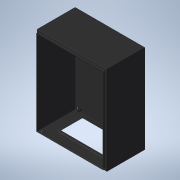
# Autodesk Inventor part: 1376.000(1)_P1
Saved by Autodesk Inventor 2021 (Build 250183000, 183)
## iProperties
Created: 2025-05-05
Part Number: 1376.000(1)_P1
Material: Generic
Catalog Web Link: www.cadenas.de
Description: AE 2.0 Gehaeuse-AE 2.0 Gehaeuse
Vendor: RITTAL
Document SubType Name: Modeling
Designer: psAdmin
Manufacturer: RITTAL
Mass: 2076.7 g
Surface Area: 27588 cm^2
Volume: 2076.7 cm^3
Density: 1 g/cm^3
Appearance: PSOLRGB-175-175-175
Category: PARTsolutions
Company: RITTAL
Title: 1376.000(1)_P1
Author: Cadenas PARTsolutions
Comments: AE 2.0 Gehaeuse
PSOL_IDENT_0: {$CADENAS_DATA/23d-libs/rittal/schaltschranksys/kompakt_schaltschr/parts_ae_2_0/gehaeuse_ae_2_0.prj}
PSOL_IDENT_1: ,190 {VTYP=3D},{NB=1376.000(1)_P1},{LINA=1376.000(1)_P1},{NN=AE 2.0 Gehaeuse},{DATE=28.04.2025 21:11
PSOL_IDENT_2: :32},{GEOMDATE=11.04.2025 11:21:47},{VERSION=},{LINEID=320},{WBVAR=DETAIL},{WBNUMERIC=DETAIL}  {NB=1
PSOL_IDENT_3: 376.000(1)_P1},{LINA=1376.000(1)_P1},{KT=DUMMY},{DETAIL=1},{BEZ1=Neues Kompaktgehäuse},{BEZ2=Stahlbl
PSOL_IDENT_4: ech},{BEZ3=eintürig},{TUER=1},{B=600},{H=760},{T=350},{F=550},{G=735},{B1=600},{BEST=1376.000},{B3=5
PSOL_IDENT_5: 60.000},{B4=372.000},{B5=400.000},{BB5=0.000},{H1=760},{H3=720.000},{H4=157.000},{H5=185.000},{HH5=4
PSOL_IDENT_6: .000},{T5=129.500},{R1=31.000},{R2=8.000},{T1=350},{F1=550},{G1=735},{VERS3=0},{VERS=1},{CNSECLASS51=
PSOL_IDENT_7: 27-18-01-02},{CNSECLASS70=27-18-01-01},{CNSECLASS80=27-18-01-01},{CNSETIM40=EC000261},{S=1.50},{W=60
PSOL_IDENT_8: 0.000},{W1=556.000},{W2=500.000},{HH=760.000},{HH1=716.000},{HH2=710.000},{HH3=635.000},{D=327.500},
PSOL_IDENT_9: {D1=345.100},{VERS1=1},{GEW=34},{CNSETIM80=EC000261},{CNSETIM90=EC000261},{CNSECLASS60=27-18-01-01},
PSOL_IDENT_10: {UNSPSC=31-26-15-02}
NB: 1376.000(1)_P1
NN: AE 2.0 Gehaeuse
NT: AE 2.0 Gehaeuse
NBSYN: $BEST.($DETAIL.)_P1
LINA: 1376.000(1)_P1
CATALOG: Rittal
DETAIL: hoch
BEZ1: Neues Kompaktgehäuse
BEZ2: Stahlblech
BEZ3: eintürig
TUER: 1
B: 600
H: 760
T: 350
F: 550
G: 735
B1: 600
BEST: 1376.000
B3: 560
B4: 372
B5: 400
BB5: 0
H1: 760
H3: 720
H4: 157
H5: 185
HH5: 4
T5: 129.5
R1: 31
R2: 8
T1: 350
F1: 550
G1: 735
VERS3: 0
VERS: 1
CNSECLASS70: 27-18-01-01
CNSECLASS80: 27-18-01-01
S: 1.5
W: 600
W1: 556
W2: 500
HH: 760
HH1: 716
HH2: 710
HH3: 635
D: 327.5
D1: 345.1
VERS1: 1
GEW: 34
CNSETIM80: EC000261
CNSETIM90: EC000261
CNSECLASS60: 27-18-01-01
UNSPSC: 31-26-15-02
SUPPLIER: RITTAL
ARTICLENO: 1376.000(1)_P1
BOMINFO: 1376.000(1)_P1
CREATOR: CADENAS GmbH
Autodesk Inventor part; units mm, degrees
(part 1 of 2)
sketch "Sketch_1" plane through (0, 0, 0) normal (0, 1, 0) x (1, 0, 0)
  line L0 (-300, -152.5) -> (300, -152.5)
  line L1 (300, -152.5) -> (300, 175)
  line L2 (300, 175) -> (-300, 175)
  line L3 (-300, 175) -> (-300, -152.5)
  arc A0 (-298.5, -149.5) -> (-297, -151) centre (-297, -149.5) ccw
  line L4 (-297, -151) -> (297, -151)
  arc A1 (297, -151) -> (298.5, -149.5) centre (297, -149.5) ccw
  line L5 (298.5, -149.5) -> (298.5, 172)
  arc A2 (298.5, 172) -> (297, 173.5) centre (297, 172) ccw
  line L6 (297, 173.5) -> (-297, 173.5)
  arc A3 (-297, 173.5) -> (-298.5, 172) centre (-297, 172) ccw
  line L7 (-298.5, 172) -> (-298.5, -149.5)
  constraints: 16 end point, 8 point on circle, 4 centre point
extrude "Extrusion1" add sketch "Sketch_1" along normal blind 760
sketch "Sketch_2" plane through (0, 0, 152.5) normal (0, 0, 1) x (1, 0, 0)
  line L0 (-281, 19) -> (281, 19)
  line L1 (281, 19) -> (281, 741)
  line L2 (281, 741) -> (-281, 741)
  line L3 (-281, 741) -> (-281, 19)
  constraints: 8 end point
extrude "Extrusion2" cut sketch "Sketch_2" against normal blind 1.5
sketch "Sketch_3" plane through (0, 0, 0) normal (1, 0, 0) x (0, 0, -1)
  line L0 (-152.5, 750) -> (-151, 750)
  line L1 (-151, 750) -> (-151, 757)
  arc A0 (-149.5, 758.5) -> (-151, 757) centre (-149.5, 757) ccw
  line L2 (-149.5, 758.5) -> (172, 758.5)
  arc A1 (173.5, 757) -> (172, 758.5) centre (172, 757) ccw
  line L3 (173.5, 757) -> (173.5, 3)
  arc A2 (172, 1.5) -> (173.5, 3) centre (172, 3) ccw
  line L4 (172, 1.5) -> (-149.5, 1.5)
  arc A3 (-151, 3) -> (-149.5, 1.5) centre (-149.5, 3) ccw
  line L5 (-151, 3) -> (-151, 10)
  line L6 (-151, 10) -> (-152.5, 10)
  line L7 (-152.5, 10) -> (-152.5, 0)
  line L8 (-152.5, 0) -> (175, 0)
  line L9 (175, 0) -> (175, 760)
  line L10 (175, 760) -> (-152.5, 760)
  line L11 (-152.5, 760) -> (-152.5, 750)
  constraints: 24 end point, 8 point on circle, 4 centre point
extrude "Extrusion3" add sketch "Sketch_3" along normal mid plane 600
sketch "Sketch_4" plane through (0, 0, 0) normal (1, 0, 0) x (0, 0, -1)
  line L0 (-154, 761.5) -> (-154, -1.5)
  line L1 (-154, -1.5) -> (176.5, -1.5)
  line L2 (176.5, -1.5) -> (176.5, 761.5)
  line L3 (176.5, 761.5) -> (-154, 761.5)
  line L4 (-152.5, 757) -> (-152.5, 3)
  arc A0 (-152.5, 3) -> (-149.5, 0) centre (-149.5, 3) ccw
  line L5 (-149.5, 0) -> (172, 0)
  arc A1 (172, 0) -> (175, 3) centre (172, 3) ccw
  line L6 (175, 3) -> (175, 757)
  arc A2 (175, 757) -> (172, 760) centre (172, 757) ccw
  line L7 (172, 760) -> (-149.5, 760)
  arc A3 (-149.5, 760) -> (-152.5, 757) centre (-149.5, 757) ccw
  constraints: 16 end point, 8 point on circle, 4 centre point
extrude "Extrusion4" cut sketch "Sketch_4" along normal mid plane 600
sketch "Sketch_5" plane through (0, 0, 0) normal (0, 1, 0) x (1, 0, 0)
  line L0 (-301.5, -154) -> (301.5, -154)
  line L1 (301.5, -154) -> (301.5, 176.5)
  line L2 (301.5, 176.5) -> (-301.5, 176.5)
  line L3 (-301.5, 176.5) -> (-301.5, -154)
  arc A0 (-300, -149.5) -> (-297, -152.5) centre (-297, -149.5) ccw
  line L4 (-297, -152.5) -> (297, -152.5)
  arc A1 (297, -152.5) -> (300, -149.5) centre (297, -149.5) ccw
  line L5 (300, -149.5) -> (300, 172)
  arc A2 (300, 172) -> (297, 175) centre (297, 172) ccw
  line L6 (297, 175) -> (-297, 175)
  arc A3 (-297, 175) -> (-300, 172) centre (-297, 172) ccw
  line L7 (-300, 172) -> (-300, -149.5)
  constraints: 16 end point, 8 point on circle, 4 centre point
extrude "Extrusion5" cut sketch "Sketch_5" along normal blind 760
sketch "Sketch_48" plane through (0, 0, -175) normal (0, 0, 1) x (1, 0, 0)
  line L0 (-295.5, 755.5) -> (-295.5, 4.5)
  line L1 (-295.5, 4.5) -> (295.5, 4.5)
  line L2 (295.5, 4.5) -> (295.5, 755.5)
  line L3 (295.5, 755.5) -> (-295.5, 755.5)
  constraints: 8 end point
extrude "Extrusion6" cut sketch "Sketch_48" along normal blind 1.5
sketch "Sketch_49" plane through (0, 0, -175) normal (0, 0, 1) x (1, 0, 0)
  line L0 (-295.5, 755.5) -> (-295.5, 4.5)
  line L1 (-295.5, 4.5) -> (295.5, 4.5)
  line L2 (295.5, 4.5) -> (295.5, 755.5)
  line L3 (295.5, 755.5) -> (-295.5, 755.5)
  line L4 (268.5, 8.5) -> (291.5, 8.5)
  line L5 (291.5, 8.5) -> (291.5, 31.5)
  line L6 (291.5, 31.5) -> (268.5, 31.5)
  line L7 (268.5, 31.5) -> (268.5, 8.5)
  line L8 (268.5, 728.5) -> (291.5, 728.5)
  line L9 (291.5, 728.5) -> (291.5, 751.5)
  line L10 (291.5, 751.5) -> (268.5, 751.5)
  line L11 (268.5, 751.5) -> (268.5, 728.5)
  line L12 (-291.5, 8.5) -> (-268.5, 8.5)
  line L13 (-268.5, 8.5) -> (-268.5, 31.5)
  line L14 (-268.5, 31.5) -> (-291.5, 31.5)
  line L15 (-291.5, 31.5) -> (-291.5, 8.5)
  line L16 (-291.5, 728.5) -> (-268.5, 728.5)
  line L17 (-268.5, 728.5) -> (-268.5, 751.5)
  line L18 (-268.5, 751.5) -> (-291.5, 751.5)
  line L19 (-291.5, 751.5) -> (-291.5, 728.5)
  constraints: 40 end point
extrude "Extrusion7" add sketch "Sketch_49" along normal blind 1.5
sketch "Sketch_105" plane through (0, 0, -175) normal (0, 0, 1) x (1, 0, 0)
  line L0 (-320, 780) -> (-320, -20)
  line L1 (-320, -20) -> (320, -20)
  line L2 (320, -20) -> (320, 780)
  line L3 (320, 780) -> (-320, 780)
  line L4 (-300, 757) -> (-300, 3)
  arc A0 (-300, 3) -> (-297, 0) centre (-297, 3) ccw
  line L5 (-297, 0) -> (297, 0)
  arc A1 (297, 0) -> (300, 3) centre (297, 3) ccw
  line L6 (300, 3) -> (300, 757)
  arc A2 (300, 757) -> (297, 760) centre (297, 757) ccw
  line L7 (297, 760) -> (-297, 760)
  arc A3 (-297, 760) -> (-300, 757) centre (-297, 757) ccw
  constraints: 16 end point, 8 point on circle, 4 centre point
extrude "Extrusion8" cut sketch "Sketch_105" along normal blind 350
sketch "Sketch_50" plane through (0, 20, 0) normal (0, 1, 0) x (1, 0, 0)
  line L0 (-291.5, 173.5) -> (-290.1732, 173.5)
  line L1 (-290.1732, 173.5) -> (-289.0185, 171.5)
  line L2 (-289.0185, 171.5) -> (-270.9815, 171.5)
  line L3 (-270.9815, 171.5) -> (-269.8268, 173.5)
  line L4 (-269.8268, 173.5) -> (-268.5, 173.5)
  line L5 (-268.5, 173.5) -> (-268.5, 175)
  line L6 (-268.5, 175) -> (-270, 175)
  line L7 (-270, 175) -> (-271.1547, 173)
  line L8 (-271.1547, 173) -> (-288.8453, 173)
  line L9 (-288.8453, 173) -> (-290, 175)
  line L10 (-290, 175) -> (-291.5, 175)
  line L11 (-291.5, 175) -> (-291.5, 173.5)
  constraints: 24 end point
extrude "Extrusion9" add sketch "Sketch_50" along normal mid plane 15.35
sketch "Sketch_51" plane through (0, 20, 0) normal (0, 1, 0) x (1, 0, 0)
  line L0 (268.5, 173.5) -> (269.8268, 173.5)
  line L1 (269.8268, 173.5) -> (270.9815, 171.5)
  line L2 (270.9815, 171.5) -> (289.0185, 171.5)
  line L3 (289.0185, 171.5) -> (290.1732, 173.5)
  line L4 (290.1732, 173.5) -> (291.5, 173.5)
  line L5 (291.5, 173.5) -> (291.5, 175)
  line L6 (291.5, 175) -> (290, 175)
  line L7 (290, 175) -> (288.8453, 173)
  line L8 (288.8453, 173) -> (271.1547, 173)
  line L9 (271.1547, 173) -> (270, 175)
  line L10 (270, 175) -> (268.5, 175)
  line L11 (268.5, 175) -> (268.5, 173.5)
  constraints: 24 end point
extrude "Extrusion10" add sketch "Sketch_51" along normal mid plane 15.35
sketch "Sketch_52" plane through (0, 27.675, 0) normal (0, 1, 0) x (1, 0, 0)
  line L0 (-272.325, 171.5) -> (-272.325, 173)
  line L1 (-272.325, 173) -> (-271.1547, 173)
  line L2 (-271.1547, 173) -> (-270, 175)
  line L3 (-270, 175) -> (-265.5, 175)
  line L4 (-265.5, 175) -> (-265.5, 173.5)
  line L5 (-265.5, 173.5) -> (-269.8268, 173.5)
  line L6 (-269.8268, 173.5) -> (-270.9815, 171.5)
  line L7 (-270.9815, 171.5) -> (-272.325, 171.5)
  line L8 (-272.325, 171.5) -> (-272.325, 173)
  constraints: 18 end point
revolve "Revolution1" add sketch "Sketch_52" angle 90 about axis through (-272.325, 27.675, -171.5) along (0, 0, 1)
sketch "Sketch_53" plane through (0, 27.675, 0) normal (0, 1, 0) x (1, 0, 0)
  line L0 (-287.675, 173) -> (-287.675, 171.5)
  line L1 (-287.675, 171.5) -> (-289.0185, 171.5)
  line L2 (-289.0185, 171.5) -> (-290.1732, 173.5)
  line L3 (-290.1732, 173.5) -> (-294.5, 173.5)
  line L4 (-294.5, 173.5) -> (-294.5, 175)
  line L5 (-294.5, 175) -> (-290, 175)
  line L6 (-290, 175) -> (-288.8453, 173)
  line L7 (-288.8453, 173) -> (-287.675, 173)
  line L8 (-287.675, 173) -> (-287.675, 171.5)
  constraints: 18 end point
revolve "Revolution2" add sketch "Sketch_53" angle 90 about axis through (-287.675, 27.675, -173) along (0, 0, -1)
sketch "Sketch_54" plane through (0, 27.675, 0) normal (0, 1, 0) x (1, 0, 0)
  line L0 (287.675, 171.5) -> (287.675, 173)
  line L1 (287.675, 173) -> (288.8453, 173)
  line L2 (288.8453, 173) -> (290, 175)
  line L3 (290, 175) -> (294.5, 175)
  line L4 (294.5, 175) -> (294.5, 173.5)
  line L5 (294.5, 173.5) -> (290.1732, 173.5)
  line L6 (290.1732, 173.5) -> (289.0185, 171.5)
  line L7 (289.0185, 171.5) -> (287.675, 171.5)
  line L8 (287.675, 171.5) -> (287.675, 173)
  constraints: 18 end point
revolve "Revolution3" add sketch "Sketch_54" angle 90 about axis through (287.675, 27.675, -171.5) along (0, 0, 1)
sketch "Sketch_55" plane through (0, 27.675, 0) normal (0, 1, 0) x (1, 0, 0)
  line L0 (272.325, 173) -> (272.325, 171.5)
  line L1 (272.325, 171.5) -> (270.9815, 171.5)
  line L2 (270.9815, 171.5) -> (269.8268, 173.5)
  line L3 (269.8268, 173.5) -> (265.5, 173.5)
  line L4 (265.5, 173.5) -> (265.5, 175)
  line L5 (265.5, 175) -> (270, 175)
  line L6 (270, 175) -> (271.1547, 173)
  line L7 (271.1547, 173) -> (272.325, 173)
  line L8 (272.325, 173) -> (272.325, 171.5)
  constraints: 18 end point
revolve "Revolution4" add sketch "Sketch_55" angle 90 about axis through (272.325, 27.675, -173) along (0, 0, -1)
sketch "Sketch_56" plane through (0, 12.325, 0) normal (0, 1, 0) x (1, 0, 0)
  line L0 (-272.325, 171.5) -> (-272.325, 173)
  line L1 (-272.325, 173) -> (-271.1547, 173)
  line L2 (-271.1547, 173) -> (-270, 175)
  line L3 (-270, 175) -> (-265.5, 175)
  line L4 (-265.5, 175) -> (-265.5, 173.5)
  line L5 (-265.5, 173.5) -> (-269.8268, 173.5)
  line L6 (-269.8268, 173.5) -> (-270.9815, 171.5)
  line L7 (-270.9815, 171.5) -> (-272.325, 171.5)
  line L8 (-272.325, 171.5) -> (-272.325, 173)
  constraints: 18 end point
revolve "Revolution5" add sketch "Sketch_56" angle 90 about axis through (-272.325, 12.325, -171.5) along (0, 0, -1)
sketch "Sketch_57" plane through (0, 12.325, 0) normal (0, 1, 0) x (1, 0, 0)
  line L0 (-287.675, 173) -> (-287.675, 171.5)
  line L1 (-287.675, 171.5) -> (-289.0185, 171.5)
  line L2 (-289.0185, 171.5) -> (-290.1732, 173.5)
  line L3 (-290.1732, 173.5) -> (-294.5, 173.5)
  line L4 (-294.5, 173.5) -> (-294.5, 175)
  line L5 (-294.5, 175) -> (-290, 175)
  line L6 (-290, 175) -> (-288.8453, 173)
  line L7 (-288.8453, 173) -> (-287.675, 173)
  line L8 (-287.675, 173) -> (-287.675, 171.5)
  constraints: 18 end point
revolve "Revolution6" add sketch "Sketch_57" angle 90 about axis through (-287.675, 12.325, -173) along (0, 0, 1)
sketch "Sketch_58" plane through (0, 12.325, 0) normal (0, 1, 0) x (1, 0, 0)
  line L0 (287.675, 171.5) -> (287.675, 173)
  line L1 (287.675, 173) -> (288.8453, 173)
  line L2 (288.8453, 173) -> (290, 175)
  line L3 (290, 175) -> (294.5, 175)
  line L4 (294.5, 175) -> (294.5, 173.5)
  line L5 (294.5, 173.5) -> (290.1732, 173.5)
  line L6 (290.1732, 173.5) -> (289.0185, 171.5)
  line L7 (289.0185, 171.5) -> (287.675, 171.5)
  line L8 (287.675, 171.5) -> (287.675, 173)
  constraints: 18 end point
revolve "Revolution7" add sketch "Sketch_58" angle 90 about axis through (287.675, 12.325, -171.5) along (0, 0, -1)
sketch "Sketch_59" plane through (0, 12.325, 0) normal (0, 1, 0) x (1, 0, 0)
  line L0 (272.325, 173) -> (272.325, 171.5)
  line L1 (272.325, 171.5) -> (270.9815, 171.5)
  line L2 (270.9815, 171.5) -> (269.8268, 173.5)
  line L3 (269.8268, 173.5) -> (265.5, 173.5)
  line L4 (265.5, 173.5) -> (265.5, 175)
  line L5 (265.5, 175) -> (270, 175)
  line L6 (270, 175) -> (271.1547, 173)
  line L7 (271.1547, 173) -> (272.325, 173)
  line L8 (272.325, 173) -> (272.325, 171.5)
  constraints: 18 end point
revolve "Revolution8" add sketch "Sketch_59" angle 90 about axis through (272.325, 12.325, -173) along (0, 0, 1)
sketch "Sketch_60" plane through (0, 740, 0) normal (0, 1, 0) x (1, 0, 0)
  line L0 (-291.5, 173.5) -> (-290.1732, 173.5)
  line L1 (-290.1732, 173.5) -> (-289.0185, 171.5)
  line L2 (-289.0185, 171.5) -> (-270.9815, 171.5)
  line L3 (-270.9815, 171.5) -> (-269.8268, 173.5)
  line L4 (-269.8268, 173.5) -> (-268.5, 173.5)
  line L5 (-268.5, 173.5) -> (-268.5, 175)
  line L6 (-268.5, 175) -> (-270, 175)
  line L7 (-270, 175) -> (-271.1547, 173)
  line L8 (-271.1547, 173) -> (-288.8453, 173)
  line L9 (-288.8453, 173) -> (-290, 175)
  line L10 (-290, 175) -> (-291.5, 175)
  line L11 (-291.5, 175) -> (-291.5, 173.5)
  constraints: 24 end point
extrude "Extrusion11" add sketch "Sketch_60" along normal mid plane 15.35
sketch "Sketch_61" plane through (0, 740, 0) normal (0, 1, 0) x (1, 0, 0)
  line L0 (268.5, 173.5) -> (269.8268, 173.5)
  line L1 (269.8268, 173.5) -> (270.9815, 171.5)
  line L2 (270.9815, 171.5) -> (289.0185, 171.5)
  line L3 (289.0185, 171.5) -> (290.1732, 173.5)
  line L4 (290.1732, 173.5) -> (291.5, 173.5)
  line L5 (291.5, 173.5) -> (291.5, 175)
  line L6 (291.5, 175) -> (290, 175)
  line L7 (290, 175) -> (288.8453, 173)
  line L8 (288.8453, 173) -> (271.1547, 173)
  line L9 (271.1547, 173) -> (270, 175)
  line L10 (270, 175) -> (268.5, 175)
  line L11 (268.5, 175) -> (268.5, 173.5)
  constraints: 24 end point
extrude "Extrusion12" add sketch "Sketch_61" along normal mid plane 15.35
sketch "Sketch_62" plane through (0, 747.675, 0) normal (0, 1, 0) x (1, 0, 0)
  line L0 (-272.325, 171.5) -> (-272.325, 173)
  line L1 (-272.325, 173) -> (-271.1547, 173)
  line L2 (-271.1547, 173) -> (-270, 175)
  line L3 (-270, 175) -> (-265.5, 175)
  line L4 (-265.5, 175) -> (-265.5, 173.5)
  line L5 (-265.5, 173.5) -> (-269.8268, 173.5)
  line L6 (-269.8268, 173.5) -> (-270.9815, 171.5)
  line L7 (-270.9815, 171.5) -> (-272.325, 171.5)
  line L8 (-272.325, 171.5) -> (-272.325, 173)
  constraints: 18 end point
revolve "Revolution9" add sketch "Sketch_62" angle 90 about axis through (-272.325, 747.675, -171.5) along (0, 0, 1)
sketch "Sketch_63" plane through (0, 747.675, 0) normal (0, 1, 0) x (1, 0, 0)
  line L0 (-287.675, 173) -> (-287.675, 171.5)
  line L1 (-287.675, 171.5) -> (-289.0185, 171.5)
  line L2 (-289.0185, 171.5) -> (-290.1732, 173.5)
  line L3 (-290.1732, 173.5) -> (-294.5, 173.5)
  line L4 (-294.5, 173.5) -> (-294.5, 175)
  line L5 (-294.5, 175) -> (-290, 175)
  line L6 (-290, 175) -> (-288.8453, 173)
  line L7 (-288.8453, 173) -> (-287.675, 173)
  line L8 (-287.675, 173) -> (-287.675, 171.5)
  constraints: 18 end point
revolve "Revolution10" add sketch "Sketch_63" angle 90 about axis through (-287.675, 747.675, -173) along (0, 0, -1)
sketch "Sketch_64" plane through (0, 747.675, 0) normal (0, 1, 0) x (1, 0, 0)
  line L0 (287.675, 171.5) -> (287.675, 173)
  line L1 (287.675, 173) -> (288.8453, 173)
  line L2 (288.8453, 173) -> (290, 175)
  line L3 (290, 175) -> (294.5, 175)
  line L4 (294.5, 175) -> (294.5, 173.5)
  line L5 (294.5, 173.5) -> (290.1732, 173.5)
  line L6 (290.1732, 173.5) -> (289.0185, 171.5)
  line L7 (289.0185, 171.5) -> (287.675, 171.5)
  line L8 (287.675, 171.5) -> (287.675, 173)
  constraints: 18 end point
revolve "Revolution11" add sketch "Sketch_64" angle 90 about axis through (287.675, 747.675, -171.5) along (0, 0, 1)
sketch "Sketch_65" plane through (0, 747.675, 0) normal (0, 1, 0) x (1, 0, 0)
  line L0 (272.325, 173) -> (272.325, 171.5)
  line L1 (272.325, 171.5) -> (270.9815, 171.5)
  line L2 (270.9815, 171.5) -> (269.8268, 173.5)
  line L3 (269.8268, 173.5) -> (265.5, 173.5)
  line L4 (265.5, 173.5) -> (265.5, 175)
  line L5 (265.5, 175) -> (270, 175)
  line L6 (270, 175) -> (271.1547, 173)
  line L7 (271.1547, 173) -> (272.325, 173)
  line L8 (272.325, 173) -> (272.325, 171.5)
  constraints: 18 end point
revolve "Revolution12" add sketch "Sketch_65" angle 90 about axis through (272.325, 747.675, -173) along (0, 0, -1)
sketch "Sketch_66" plane through (0, 732.325, 0) normal (0, 1, 0) x (1, 0, 0)
  line L0 (-272.325, 171.5) -> (-272.325, 173)
  line L1 (-272.325, 173) -> (-271.1547, 173)
  line L2 (-271.1547, 173) -> (-270, 175)
  line L3 (-270, 175) -> (-265.5, 175)
  line L4 (-265.5, 175) -> (-265.5, 173.5)
  line L5 (-265.5, 173.5) -> (-269.8268, 173.5)
  line L6 (-269.8268, 173.5) -> (-270.9815, 171.5)
  line L7 (-270.9815, 171.5) -> (-272.325, 171.5)
  line L8 (-272.325, 171.5) -> (-272.325, 173)
  constraints: 18 end point
revolve "Revolution13" add sketch "Sketch_66" angle 90 about axis through (-272.325, 732.325, -171.5) along (0, 0, -1)
sketch "Sketch_67" plane through (0, 732.325, 0) normal (0, 1, 0) x (1, 0, 0)
  line L0 (-287.675, 173) -> (-287.675, 171.5)
  line L1 (-287.675, 171.5) -> (-289.0185, 171.5)
  line L2 (-289.0185, 171.5) -> (-290.1732, 173.5)
  line L3 (-290.1732, 173.5) -> (-294.5, 173.5)
  line L4 (-294.5, 173.5) -> (-294.5, 175)
  line L5 (-294.5, 175) -> (-290, 175)
  line L6 (-290, 175) -> (-288.8453, 173)
  line L7 (-288.8453, 173) -> (-287.675, 173)
  line L8 (-287.675, 173) -> (-287.675, 171.5)
  constraints: 18 end point
revolve "Revolution14" add sketch "Sketch_67" angle 90 about axis through (-287.675, 732.325, -173) along (0, 0, 1)
sketch "Sketch_68" plane through (0, 732.325, 0) normal (0, 1, 0) x (1, 0, 0)
  line L0 (287.675, 171.5) -> (287.675, 173)
  line L1 (287.675, 173) -> (288.8453, 173)
  line L2 (288.8453, 173) -> (290, 175)
  line L3 (290, 175) -> (294.5, 175)
  line L4 (294.5, 175) -> (294.5, 173.5)
  line L5 (294.5, 173.5) -> (290.1732, 173.5)
  line L6 (290.1732, 173.5) -> (289.0185, 171.5)
  line L7 (289.0185, 171.5) -> (287.675, 171.5)
  line L8 (287.675, 171.5) -> (287.675, 173)
  constraints: 18 end point
revolve "Revolution15" add sketch "Sketch_68" angle 90 about axis through (287.675, 732.325, -171.5) along (0, 0, -1)
sketch "Sketch_69" plane through (0, 732.325, 0) normal (0, 1, 0) x (1, 0, 0)
  line L0 (272.325, 173) -> (272.325, 171.5)
  line L1 (272.325, 171.5) -> (270.9815, 171.5)
  line L2 (270.9815, 171.5) -> (269.8268, 173.5)
  line L3 (269.8268, 173.5) -> (265.5, 173.5)
  line L4 (265.5, 173.5) -> (265.5, 175)
  line L5 (265.5, 175) -> (270, 175)
  line L6 (270, 175) -> (271.1547, 173)
  line L7 (271.1547, 173) -> (272.325, 173)
  line L8 (272.325, 173) -> (272.325, 171.5)
  constraints: 18 end point
revolve "Revolution16" add sketch "Sketch_69" angle 90 about axis through (272.325, 732.325, -173) along (0, 0, 1)
sketch "Sketch_70" plane through (-280, 0, 0) normal (1, 0, 0) x (0, 0, -1)
  line L0 (171.5, 10.9815) -> (173.5, 9.8268)
  line L1 (173.5, 9.8268) -> (173.5, 8.5)
  line L2 (173.5, 8.5) -> (175, 8.5)
  line L3 (175, 8.5) -> (175, 10)
  line L4 (175, 10) -> (173, 11.1547)
  line L5 (173, 11.1547) -> (173, 28.8453)
  line L6 (173, 28.8453) -> (175, 30)
  line L7 (175, 30) -> (175, 31.5)
  line L8 (175, 31.5) -> (173.5, 31.5)
  line L9 (173.5, 31.5) -> (173.5, 30.1732)
  line L10 (173.5, 30.1732) -> (171.5, 29.0185)
  line L11 (171.5, 29.0185) -> (171.5, 10.9815)
  constraints: 24 end point
extrude "Extrusion13" add sketch "Sketch_70" along normal mid plane 15.35
sketch "Sketch_71" plane through (-280, 0, 0) normal (1, 0, 0) x (0, 0, -1)
  line L0 (171.5, 730.9815) -> (173.5, 729.8268)
  line L1 (173.5, 729.8268) -> (173.5, 728.5)
  line L2 (173.5, 728.5) -> (175, 728.5)
  line L3 (175, 728.5) -> (175, 730)
  line L4 (175, 730) -> (173, 731.1547)
  line L5 (173, 731.1547) -> (173, 748.8453)
  line L6 (173, 748.8453) -> (175, 750)
  line L7 (175, 750) -> (175, 751.5)
  line L8 (175, 751.5) -> (173.5, 751.5)
  line L9 (173.5, 751.5) -> (173.5, 750.1732)
  line L10 (173.5, 750.1732) -> (171.5, 749.0185)
  line L11 (171.5, 749.0185) -> (171.5, 730.9815)
  constraints: 24 end point
extrude "Extrusion14" add sketch "Sketch_71" along normal mid plane 15.35
sketch "Sketch_74" plane through (-280, 0, 0) normal (1, 0, 0) x (0, 0, -1)
  line L0 (174.5, 20) -> (171.5, 20)
  line L1 (171.5, 20) -> (171.5, 26.25)
  line L2 (171.5, 26.25) -> (173, 26.25)
  line L3 (173, 26.25) -> (173, 25.6)
  line L4 (173, 25.6) -> (174.5, 25.6)
  line L5 (174.5, 25.6) -> (174.5, 20)
  line L6 (174.5, 20) -> (171.5, 20)
  constraints: 14 end point
revolve "Revolution17" add sketch "Sketch_74" angle 360 about axis through (-280, 20, -174.5) along (0, 0, 1)
sketch "Sketch_75" plane through (-280, 0, 0) normal (1, 0, 0) x (0, 0, -1)
  line L0 (175, 20) -> (171, 20)
  line L1 (171, 20) -> (171, 25.625)
  line L2 (171, 25.625) -> (171.5, 25.625)
  arc A0 (171.5, 25.625) -> (172.5, 24.625) centre (172.5, 25.625) ccw
  line L3 (172.5, 24.625) -> (174.3, 24.625)
  arc A1 (174.3, 24.625) -> (174.5, 24.825) centre (174.3, 24.825) ccw
  line L4 (174.5, 24.825) -> (174.5, 25.625)
  line L5 (174.5, 25.625) -> (175, 25.625)
  line L6 (175, 25.625) -> (175, 20)
  line L7 (175, 20) -> (171, 20)
  constraints: 16 end point, 4 point on circle, 2 centre point
revolve "Revolution18" cut sketch "Sketch_75" angle 360 about axis through (-280, 20, -175) along (0, 0, 1)
sketch "Sketch_76" plane through (-280, 0, 0) normal (1, 0, 0) x (0, 0, -1)
  line L0 (174.5, 740) -> (171.5, 740)
  line L1 (171.5, 740) -> (171.5, 746.25)
  line L2 (171.5, 746.25) -> (173, 746.25)
  line L3 (173, 746.25) -> (173, 745.6)
  line L4 (173, 745.6) -> (174.5, 745.6)
  line L5 (174.5, 745.6) -> (174.5, 740)
  line L6 (174.5, 740) -> (171.5, 740)
  constraints: 14 end point
revolve "Revolution19" add sketch "Sketch_76" angle 360 about axis through (-280, 740, -174.5) along (0, 0, 1)
sketch "Sketch_77" plane through (-280, 0, 0) normal (1, 0, 0) x (0, 0, -1)
  line L0 (175, 740) -> (171, 740)
  line L1 (171, 740) -> (171, 745.625)
  line L2 (171, 745.625) -> (171.5, 745.625)
  arc A0 (171.5, 745.625) -> (172.5, 744.625) centre (172.5, 745.625) ccw
  line L3 (172.5, 744.625) -> (174.3, 744.625)
  arc A1 (174.3, 744.625) -> (174.5, 744.825) centre (174.3, 744.825) ccw
  line L4 (174.5, 744.825) -> (174.5, 745.625)
  line L5 (174.5, 745.625) -> (175, 745.625)
  line L6 (175, 745.625) -> (175, 740)
  line L7 (175, 740) -> (171, 740)
  constraints: 16 end point, 4 point on circle, 2 centre point
revolve "Revolution20" cut sketch "Sketch_77" angle 360 about axis through (-280, 740, -175) along (0, 0, 1)
sketch "Sketch_72" plane through (280, 0, 0) normal (1, 0, 0) x (0, 0, -1)
  line L0 (171.5, 10.9815) -> (173.5, 9.8268)
  line L1 (173.5, 9.8268) -> (173.5, 8.5)
  line L2 (173.5, 8.5) -> (175, 8.5)
  line L3 (175, 8.5) -> (175, 10)
  line L4 (175, 10) -> (173, 11.1547)
  line L5 (173, 11.1547) -> (173, 28.8453)
  line L6 (173, 28.8453) -> (175, 30)
  line L7 (175, 30) -> (175, 31.5)
  line L8 (175, 31.5) -> (173.5, 31.5)
  line L9 (173.5, 31.5) -> (173.5, 30.1732)
  line L10 (173.5, 30.1732) -> (171.5, 29.0185)
  line L11 (171.5, 29.0185) -> (171.5, 10.9815)
  constraints: 24 end point
extrude "Extrusion15" add sketch "Sketch_72" along normal mid plane 15.35
sketch "Sketch_73" plane through (280, 0, 0) normal (1, 0, 0) x (0, 0, -1)
  line L0 (171.5, 730.9815) -> (173.5, 729.8268)
  line L1 (173.5, 729.8268) -> (173.5, 728.5)
  line L2 (173.5, 728.5) -> (175, 728.5)
  line L3 (175, 728.5) -> (175, 730)
  line L4 (175, 730) -> (173, 731.1547)
  line L5 (173, 731.1547) -> (173, 748.8453)
  line L6 (173, 748.8453) -> (175, 750)
  line L7 (175, 750) -> (175, 751.5)
  line L8 (175, 751.5) -> (173.5, 751.5)
  line L9 (173.5, 751.5) -> (173.5, 750.1732)
  line L10 (173.5, 750.1732) -> (171.5, 749.0185)
  line L11 (171.5, 749.0185) -> (171.5, 730.9815)
  constraints: 24 end point
extrude "Extrusion16" add sketch "Sketch_73" along normal mid plane 15.35
sketch "Sketch_78" plane through (280, 0, 0) normal (1, 0, 0) x (0, 0, -1)
  line L0 (174.5, 20) -> (171.5, 20)
  line L1 (171.5, 20) -> (171.5, 26.25)
  line L2 (171.5, 26.25) -> (173, 26.25)
  line L3 (173, 26.25) -> (173, 25.6)
  line L4 (173, 25.6) -> (174.5, 25.6)
  line L5 (174.5, 25.6) -> (174.5, 20)
  line L6 (174.5, 20) -> (171.5, 20)
  constraints: 14 end point
revolve "Revolution21" add sketch "Sketch_78" angle 360 about axis through (280, 20, -174.5) along (0, 0, 1)
sketch "Sketch_79" plane through (280, 0, 0) normal (1, 0, 0) x (0, 0, -1)
  line L0 (175, 20) -> (171, 20)
  line L1 (171, 20) -> (171, 25.625)
  line L2 (171, 25.625) -> (171.5, 25.625)
  arc A0 (171.5, 25.625) -> (172.5, 24.625) centre (172.5, 25.625) ccw
  line L3 (172.5, 24.625) -> (174.3, 24.625)
  arc A1 (174.3, 24.625) -> (174.5, 24.825) centre (174.3, 24.825) ccw
  line L4 (174.5, 24.825) -> (174.5, 25.625)
  line L5 (174.5, 25.625) -> (175, 25.625)
  line L6 (175, 25.625) -> (175, 20)
  line L7 (175, 20) -> (171, 20)
  constraints: 16 end point, 4 point on circle, 2 centre point
revolve "Revolution22" cut sketch "Sketch_79" angle 360 about axis through (280, 20, -175) along (0, 0, 1)
sketch "Sketch_80" plane through (280, 0, 0) normal (1, 0, 0) x (0, 0, -1)
  line L0 (174.5, 740) -> (171.5, 740)
  line L1 (171.5, 740) -> (171.5, 746.25)
  line L2 (171.5, 746.25) -> (173, 746.25)
  line L3 (173, 746.25) -> (173, 745.6)
  line L4 (173, 745.6) -> (174.5, 745.6)
  line L5 (174.5, 745.6) -> (174.5, 740)
  line L6 (174.5, 740) -> (171.5, 740)
  constraints: 14 end point
revolve "Revolution23" add sketch "Sketch_80" angle 360 about axis through (280, 740, -174.5) along (0, 0, 1)
sketch "Sketch_81" plane through (280, 0, 0) normal (1, 0, 0) x (0, 0, -1)
  line L0 (175, 740) -> (171, 740)
  line L1 (171, 740) -> (171, 745.625)
  line L2 (171, 745.625) -> (171.5, 745.625)
  arc A0 (171.5, 745.625) -> (172.5, 744.625) centre (172.5, 745.625) ccw
  line L3 (172.5, 744.625) -> (174.3, 744.625)
  arc A1 (174.3, 744.625) -> (174.5, 744.825) centre (174.3, 744.825) ccw
  line L4 (174.5, 744.825) -> (174.5, 745.625)
  line L5 (174.5, 745.625) -> (175, 745.625)
  line L6 (175, 745.625) -> (175, 740)
  line L7 (175, 740) -> (171, 740)
  constraints: 16 end point, 4 point on circle, 2 centre point
revolve "Revolution24" cut sketch "Sketch_81" angle 360 about axis through (280, 740, -175) along (0, 0, 1)
sketch "Sketch_6" plane through (0, 0, 0) normal (1, 0, 0) x (0, 0, -1)
  line L0 (-170.1, 745.9693) -> (-169.6424, 740.7385)
  arc A0 (-169.6424, 740.7385) -> (-166.6538, 738) centre (-166.6538, 741) ccw
  line L1 (-166.6538, 738) -> (-154, 738)
  arc A1 (-154, 738) -> (-151, 741) centre (-154, 741) ccw
  line L2 (-151, 741) -> (-151, 746.1)
  line L3 (-151, 746.1) -> (-168.6057, 746.1)
  line L4 (-168.6057, 746.1) -> (-170.1, 745.9693)
  constraints: 10 end point, 4 point on circle, 2 centre point
extrude "Extrusion17" add sketch "Sketch_6" along normal mid plane 574.2
sketch "Sketch_7" plane through (0, 0, 0) normal (1, 0, 0) x (0, 0, -1)
  line L0 (-170.1, 14.0307) -> (-168.6057, 13.9)
  line L1 (-168.6057, 13.9) -> (-151, 13.9)
  line L2 (-151, 13.9) -> (-151, 19)
  arc A0 (-151, 19) -> (-154, 22) centre (-154, 19) ccw
  line L3 (-154, 22) -> (-166.6538, 22)
  arc A1 (-166.6538, 22) -> (-169.6424, 19.2615) centre (-166.6538, 19) ccw
  line L4 (-169.6424, 19.2615) -> (-170.1, 14.0307)
  constraints: 10 end point, 4 point on circle, 2 centre point
extrude "Extrusion18" add sketch "Sketch_7" along normal mid plane 574.2
sketch "Sketch_8" plane through (0, 380, 0) normal (0, 1, 0) x (1, 0, 0)
  line L0 (278, -154) -> (278, -166.6538)
  arc A0 (278, -166.6538) -> (280.7385, -169.6424) centre (281, -166.6538) ccw
  line L1 (280.7385, -169.6424) -> (285.9693, -170.1)
  line L2 (285.9693, -170.1) -> (286.1, -168.6057)
  line L3 (286.1, -168.6057) -> (286.1, -151)
  line L4 (286.1, -151) -> (281, -151)
  arc A1 (281, -151) -> (278, -154) centre (281, -154) ccw
  constraints: 10 end point, 4 point on circle, 2 centre point
extrude "Extrusion19" add sketch "Sketch_8" along normal mid plane 734.2
sketch "Sketch_9" plane through (0, 380, 0) normal (0, 1, 0) x (1, 0, 0)
  line L0 (-286.1, -168.6057) -> (-285.9693, -170.1)
  line L1 (-285.9693, -170.1) -> (-280.7385, -169.6424)
  arc A0 (-280.7385, -169.6424) -> (-278, -166.6538) centre (-281, -166.6538) ccw
  line L2 (-278, -166.6538) -> (-278, -154)
  arc A1 (-278, -154) -> (-281, -151) centre (-281, -154) ccw
  line L3 (-281, -151) -> (-286.1, -151)
  line L4 (-286.1, -151) -> (-286.1, -168.6057)
  constraints: 10 end point, 4 point on circle, 2 centre point
extrude "Extrusion20" add sketch "Sketch_9" along normal mid plane 734.2
sketch "Sketch_12" plane through (0, 380, 0) normal (0, 1, 0) x (1, 0, 0)
  line L0 (-287.6, -152.5) -> (-287.6, -173.1)
  line L1 (-287.6, -173.1) -> (287.6, -173.1)
  line L2 (287.6, -173.1) -> (287.6, -152.5)
  line L3 (287.6, -152.5) -> (281, -152.5)
  arc A0 (281, -152.5) -> (279.5, -154) centre (281, -154) ccw
  line L4 (279.5, -154) -> (279.5, -166.6538)
  arc A1 (279.5, -166.6538) -> (280.8693, -168.1481) centre (281, -166.6538) ccw
  line L5 (280.8693, -168.1481) -> (286.1, -168.6057)
  line L6 (286.1, -168.6057) -> (285.9693, -170.1)
  line L7 (285.9693, -170.1) -> (-285.9693, -170.1)
  line L8 (-285.9693, -170.1) -> (-286.1, -168.6057)
  line L9 (-286.1, -168.6057) -> (-280.8693, -168.1481)
  arc A2 (-280.8693, -168.1481) -> (-279.5, -166.6538) centre (-281, -166.6538) ccw
  line L10 (-279.5, -166.6538) -> (-279.5, -154)
  arc A3 (-279.5, -154) -> (-281, -152.5) centre (-281, -154) ccw
  line L11 (-281, -152.5) -> (-287.6, -152.5)
  constraints: 24 end point, 8 point on circle, 4 centre point
extrude "Extrusion21" cut sketch "Sketch_12" along normal mid plane 732.2
sketch "Sketch_11" plane through (0, 0, 0) normal (1, 0, 0) x (0, 0, -1)
  line L0 (-173.1, 10.9) -> (-152.5, 10.9)
  line L1 (-152.5, 10.9) -> (-152.5, 19)
  arc A0 (-152.5, 19) -> (-154, 20.5) centre (-154, 19) ccw
  line L2 (-154, 20.5) -> (-166.6538, 20.5)
  arc A1 (-166.6538, 20.5) -> (-168.1481, 19.1307) centre (-166.6538, 19) ccw
  line L3 (-168.1481, 19.1307) -> (-168.6057, 13.9)
  line L4 (-168.6057, 13.9) -> (-170.1, 14.0307)
  line L5 (-170.1, 14.0307) -> (-170.1, 745.9693)
  line L6 (-170.1, 745.9693) -> (-168.6057, 746.1)
  line L7 (-168.6057, 746.1) -> (-168.1481, 740.8693)
  arc A2 (-168.1481, 740.8693) -> (-166.6538, 739.5) centre (-166.6538, 741) ccw
  line L8 (-166.6538, 739.5) -> (-154, 739.5)
  arc A3 (-154, 739.5) -> (-152.5, 741) centre (-154, 741) ccw
  line L9 (-152.5, 741) -> (-152.5, 749.1)
  line L10 (-152.5, 749.1) -> (-173.1, 749.1)
  line L11 (-173.1, 749.1) -> (-173.1, 10.9)
  constraints: 24 end point, 8 point on circle, 4 centre point
extrude "Extrusion22" cut sketch "Sketch_11" along normal mid plane 572.2
sketch "Sketch_13" plane through (0, 735, 0) normal (0, 1, 0) x (1, 0, 0)
  line L0 (-250, 142.5) -> (-250, 173.5)
  line L1 (-250, 173.5) -> (-243.5, 173.5)
  line L2 (-243.5, 173.5) -> (-243.5, 172.5)
  line L3 (-243.5, 172.5) -> (-242.45, 172.5)
  line L4 (-242.45, 172.5) -> (-242.25, 172.3)
  line L5 (-242.25, 172.3) -> (-242.25, 163.3)
  arc A0 (-242.55, 163) -> (-242.25, 163.3) centre (-242.55, 163.3) ccw
  line L6 (-242.55, 163) -> (-242.25, 163)
  line L7 (-242.25, 163) -> (-242.25, 157.5)
  line L8 (-242.25, 157.5) -> (-246, 157.5)
  line L9 (-246, 157.5) -> (-246, 155)
  line L10 (-246, 155) -> (-241, 155)
  arc A1 (-240.8875, 152.5051) -> (-241, 155) centre (-241, 153.75) ccw
  line L11 (-240.8875, 152.5051) -> (-242.2, 152.3864)
  line L12 (-242.2, 152.3864) -> (-242.2, 147.3483)
  line L13 (-242.2, 147.3483) -> (-243.5, 147)
  line L14 (-243.5, 147) -> (-246, 147)
  line L15 (-246, 147) -> (-246, 143.267)
  line L16 (-246, 143.267) -> (-246.767, 142.5)
  line L17 (-246.767, 142.5) -> (-250, 142.5)
  line L18 (-250, 142.5) -> (-250, 173.5)
  constraints: 38 end point, 4 point on circle, 2 centre point
revolve "Revolution25" add sketch "Sketch_13" angle 360 about axis through (-250, 735, -142.5) along (0, 0, 1)
thread "Thread1" size "M8x1.25" class "6g" standard "ISO Metric profile" length 1.1716
sketch "Sketch_14" plane through (0, 735, 0) normal (0, 1, 0) x (1, 0, 0)
  line L0 (250, 142.5) -> (250, 173.5)
  line L1 (250, 173.5) -> (256.5, 173.5)
  line L2 (256.5, 173.5) -> (256.5, 172.5)
  line L3 (256.5, 172.5) -> (257.55, 172.5)
  line L4 (257.55, 172.5) -> (257.75, 172.3)
  line L5 (257.75, 172.3) -> (257.75, 163.3)
  arc A0 (257.45, 163) -> (257.75, 163.3) centre (257.45, 163.3) ccw
  line L6 (257.45, 163) -> (257.75, 163)
  line L7 (257.75, 163) -> (257.75, 157.5)
  line L8 (257.75, 157.5) -> (254, 157.5)
  line L9 (254, 157.5) -> (254, 155)
  line L10 (254, 155) -> (259, 155)
  arc A1 (259.1125, 152.5051) -> (259, 155) centre (259, 153.75) ccw
  line L11 (259.1125, 152.5051) -> (257.8, 152.3864)
  line L12 (257.8, 152.3864) -> (257.8, 147.3483)
  line L13 (257.8, 147.3483) -> (256.5, 147)
  line L14 (256.5, 147) -> (254, 147)
  line L15 (254, 147) -> (254, 143.267)
  line L16 (254, 143.267) -> (253.233, 142.5)
  line L17 (253.233, 142.5) -> (250, 142.5)
  line L18 (250, 142.5) -> (250, 173.5)
  constraints: 38 end point, 4 point on circle, 2 centre point
revolve "Revolution26" add sketch "Sketch_14" angle 360 about axis through (250, 735, -142.5) along (0, 0, 1)
thread "Thread2" size "M8x1.25" class "6g" standard "ISO Metric profile" length 1.1716
sketch "Sketch_15" plane through (0, 25, 0) normal (0, 1, 0) x (1, 0, 0)
  line L0 (-250, 142.5) -> (-250, 173.5)
  line L1 (-250, 173.5) -> (-243.5, 173.5)
  line L2 (-243.5, 173.5) -> (-243.5, 172.5)
  line L3 (-243.5, 172.5) -> (-242.45, 172.5)
  line L4 (-242.45, 172.5) -> (-242.25, 172.3)
  line L5 (-242.25, 172.3) -> (-242.25, 163.3)
  arc A0 (-242.55, 163) -> (-242.25, 163.3) centre (-242.55, 163.3) ccw
  line L6 (-242.55, 163) -> (-242.25, 163)
  line L7 (-242.25, 163) -> (-242.25, 157.5)
  line L8 (-242.25, 157.5) -> (-246, 157.5)
  line L9 (-246, 157.5) -> (-246, 155)
  line L10 (-246, 155) -> (-241, 155)
  arc A1 (-240.8875, 152.5051) -> (-241, 155) centre (-241, 153.75) ccw
  line L11 (-240.8875, 152.5051) -> (-242.2, 152.3864)
  line L12 (-242.2, 152.3864) -> (-242.2, 147.3483)
  line L13 (-242.2, 147.3483) -> (-243.5, 147)
  line L14 (-243.5, 147) -> (-246, 147)
  line L15 (-246, 147) -> (-246, 143.267)
  line L16 (-246, 143.267) -> (-246.767, 142.5)
  line L17 (-246.767, 142.5) -> (-250, 142.5)
  line L18 (-250, 142.5) -> (-250, 173.5)
  constraints: 38 end point, 4 point on circle, 2 centre point
revolve "Revolution27" add sketch "Sketch_15" angle 360 about axis through (-250, 25, -142.5) along (0, 0, 1)
thread "Thread3" size "M8x1.25" class "6g" standard "ISO Metric profile" length 1.1716
sketch "Sketch_16" plane through (0, 25, 0) normal (0, 1, 0) x (1, 0, 0)
  line L0 (250, 142.5) -> (250, 173.5)
  line L1 (250, 173.5) -> (256.5, 173.5)
  line L2 (256.5, 173.5) -> (256.5, 172.5)
  line L3 (256.5, 172.5) -> (257.55, 172.5)
  line L4 (257.55, 172.5) -> (257.75, 172.3)
  line L5 (257.75, 172.3) -> (257.75, 163.3)
  arc A0 (257.45, 163) -> (257.75, 163.3) centre (257.45, 163.3) ccw
  line L6 (257.45, 163) -> (257.75, 163)
  line L7 (257.75, 163) -> (257.75, 157.5)
  line L8 (257.75, 157.5) -> (254, 157.5)
  line L9 (254, 157.5) -> (254, 155)
  line L10 (254, 155) -> (259, 155)
  arc A1 (259.1125, 152.5051) -> (259, 155) centre (259, 153.75) ccw
  line L11 (259.1125, 152.5051) -> (257.8, 152.3864)
  line L12 (257.8, 152.3864) -> (257.8, 147.3483)
  line L13 (257.8, 147.3483) -> (256.5, 147)
  line L14 (256.5, 147) -> (254, 147)
  line L15 (254, 147) -> (254, 143.267)
  line L16 (254, 143.267) -> (253.233, 142.5)
  line L17 (253.233, 142.5) -> (250, 142.5)
  line L18 (250, 142.5) -> (250, 173.5)
  constraints: 38 end point, 4 point on circle, 2 centre point
revolve "Revolution28" add sketch "Sketch_16" angle 360 about axis through (250, 25, -142.5) along (0, 0, 1)
thread "Thread4" size "M8x1.25" class "6g" standard "ISO Metric profile" length 1.1716
sketch "Sketch_100" plane through (0, 0, -146.75) normal (0, 0, 1) x (1, 0, 0)
  line L0 (-297, 757) -> (-297, 3)
  line L1 (-297, 3) -> (297, 3)
  line L2 (297, 3) -> (297, 757)
  line L3 (297, 757) -> (-297, 757)
  line L4 (243.5, 731.2472) -> (250, 727.4944)
  line L5 (250, 727.4944) -> (256.5, 731.2472)
  line L6 (256.5, 731.2472) -> (256.5, 738.7528)
  line L7 (256.5, 738.7528) -> (250, 742.5056)
  line L8 (250, 742.5056) -> (243.5, 738.7528)
  line L9 (243.5, 738.7528) -> (243.5, 731.2472)
  line L10 (243.5, 21.2472) -> (250, 17.4944)
  line L11 (250, 17.4944) -> (256.5, 21.2472)
  line L12 (256.5, 21.2472) -> (256.5, 28.7528)
  line L13 (256.5, 28.7528) -> (250, 32.5056)
  line L14 (250, 32.5056) -> (243.5, 28.7528)
  line L15 (243.5, 28.7528) -> (243.5, 21.2472)
  line L16 (-6.5, 731.2472) -> (0, 727.4944)
  line L17 (0, 727.4944) -> (6.5, 731.2472)
  line L18 (6.5, 731.2472) -> (6.5, 738.7528)
  line L19 (6.5, 738.7528) -> (0, 742.5056)
  line L20 (0, 742.5056) -> (-6.5, 738.7528)
  line L21 (-6.5, 738.7528) -> (-6.5, 731.2472)
  line L22 (-6.5, 21.2472) -> (0, 17.4944)
  line L23 (0, 17.4944) -> (6.5, 21.2472)
  line L24 (6.5, 21.2472) -> (6.5, 28.7528)
  line L25 (6.5, 28.7528) -> (0, 32.5056)
  line L26 (0, 32.5056) -> (-6.5, 28.7528)
  line L27 (-6.5, 28.7528) -> (-6.5, 21.2472)
  line L28 (-256.5, 731.2472) -> (-250, 727.4944)
  line L29 (-250, 727.4944) -> (-243.5, 731.2472)
  line L30 (-243.5, 731.2472) -> (-243.5, 738.7528)
  line L31 (-243.5, 738.7528) -> (-250, 742.5056)
  line L32 (-250, 742.5056) -> (-256.5, 738.7528)
  line L33 (-256.5, 738.7528) -> (-256.5, 731.2472)
  line L34 (-256.5, 21.2472) -> (-250, 17.4944)
  line L35 (-250, 17.4944) -> (-243.5, 21.2472)
  line L36 (-243.5, 21.2472) -> (-243.5, 28.7528)
  line L37 (-243.5, 28.7528) -> (-250, 32.5056)
  line L38 (-250, 32.5056) -> (-256.5, 28.7528)
  line L39 (-256.5, 28.7528) -> (-256.5, 21.2472)
  constraints: 80 end point
extrude "Extrusion23" cut sketch "Sketch_100" against normal blind 6
sketch "Sketch_139" plane through (0, 25, 0) normal (0, 1, 0) x (1, 0, 0)
  line L0 (-250, 151.6814) -> (-250, 155)
  line L1 (-250, 155) -> (-241, 155)
  arc A0 (-240.8875, 152.5051) -> (-241, 155) centre (-241, 153.75) ccw
  line L2 (-240.8875, 152.5051) -> (-250, 151.6814)
  line L3 (-250, 151.6814) -> (-250, 155)
  constraints: 8 end point, 2 point on circle, 1 centre point
revolve "Revolution29" add sketch "Sketch_139" angle 360 about axis through (-250, 25, -151.6814) along (0, 0, 1)
sketch "Sketch_140" plane through (0, 25, 0) normal (0, 1, 0) x (1, 0, 0)
  line L0 (250, 151.6814) -> (250, 155)
  line L1 (250, 155) -> (259, 155)
  arc A0 (259.1125, 152.5051) -> (259, 155) centre (259, 153.75) ccw
  line L2 (259.1125, 152.5051) -> (250, 151.6814)
  line L3 (250, 151.6814) -> (250, 155)
  constraints: 8 end point, 2 point on circle, 1 centre point
revolve "Revolution30" add sketch "Sketch_140" angle 360 about axis through (250, 25, -151.6814) along (0, 0, 1)
sketch "Sketch54" plane through (279.5, 20.5, 166.6538) normal (1, 0, 0) x (0, 0, -1)
  point P0 (6.9038, 677)
hole "Hole1" at (279.5, 697.5, 159.75) direction (-1, 0, 0) diameter 6.5 depth 1.5
sketch "Sketch55" plane through (279.5, 20.5, 166.6538) normal (1, 0, 0) x (0, 0, -1)
  point P0 (6.9038, 42)
hole "Hole2" at (279.5, 62.5, 159.75) direction (-1, 0, 0) diameter 6.5 depth 1.5
sketch "Sketch56" plane through (-279.5, 20.5, 154) normal (-1, 0, 0) x (0, 0, 1)
  point P0 (5.75, 677)
hole "Hole3" at (-279.5, 697.5, 159.75) direction (1, 0, 0) diameter 6.5 depth 1.5
sketch "Sketch57" plane through (-279.5, 20.5, 154) normal (-1, 0, 0) x (0, 0, 1)
  point P0 (5.75, 42)
hole "Hole4" at (-279.5, 62.5, 159.75) direction (1, 0, 0) diameter 6.5 depth 1.5
sketch "Sketch_27" plane through (0, 0, 0) normal (0, 1, 0) x (1, 0, 0)
  line L0 (-295.5, -148) -> (295.5, -148)
  line L1 (295.5, -148) -> (295.5, 170.5)
  line L2 (295.5, 170.5) -> (-295.5, 170.5)
  line L3 (-295.5, 170.5) -> (-295.5, -148)
  constraints: 8 end point
extrude "Extrusion24" cut sketch "Sketch_27" along normal blind 1.5
sketch "Sketch_28" plane through (0, 0, 0) normal (0, 1, 0) x (1, 0, 0)
  line L0 (-295.5, -148) -> (295.5, -148)
  line L1 (295.5, -148) -> (295.5, 170.5)
  line L2 (295.5, 170.5) -> (-295.5, 170.5)
  line L3 (-295.5, 170.5) -> (-295.5, -148)
  arc A0 (-225, -33) -> (-186, -72) centre (-186, -33) ccw
  line L4 (-186, -72) -> (186, -72)
  arc A1 (186, -72) -> (225, -33) centre (186, -33) ccw
  line L5 (225, -33) -> (225, 124)
  arc A2 (225, 124) -> (186, 163) centre (186, 124) ccw
  line L6 (186, 163) -> (-186, 163)
  arc A3 (-186, 163) -> (-225, 124) centre (-186, 124) ccw
  line L7 (-225, 124) -> (-225, -33)
  circle A4 centre (-283.5, -136) radius 8
  constraints: 16 end point, 8 point on circle, 5 centre point
extrude "Extrusion25" add sketch "Sketch_28" along normal blind 1.5
sketch "Sketch_29" plane through (0, 0, 0) normal (1, 0, 0) x (0, 0, -1)
  line L0 (138, 4) -> (154.5981, 4)
  line L1 (154.5981, 4) -> (161.5263, 0)
  line L2 (161.5263, 0) -> (163, 0)
  line L3 (163, 0) -> (163, 1.5)
  line L4 (163, 1.5) -> (161.9282, 1.5)
  line L5 (161.9282, 1.5) -> (155, 5.5)
  line L6 (155, 5.5) -> (138, 5.5)
  line L7 (138, 5.5) -> (138, 4)
  constraints: 16 end point
extrude "Extrusion26" add sketch "Sketch_29" along normal mid plane 372
sketch "Sketch_30" plane through (0, 0, 0) normal (1, 0, 0) x (0, 0, -1)
  line L0 (-72, 0) -> (-70.5263, 0)
  line L1 (-70.5263, 0) -> (-63.5981, 4)
  line L2 (-63.5981, 4) -> (-47, 4)
  line L3 (-47, 4) -> (-47, 5.5)
  line L4 (-47, 5.5) -> (-64, 5.5)
  line L5 (-64, 5.5) -> (-70.9282, 1.5)
  line L6 (-70.9282, 1.5) -> (-72, 1.5)
  line L7 (-72, 1.5) -> (-72, 0)
  constraints: 16 end point
extrude "Extrusion27" add sketch "Sketch_30" along normal mid plane 372
sketch "Sketch_31" plane through (186, 0, 0) normal (1, 0, 0) x (0, 0, -1)
  line L0 (124, 4) -> (124, 5.5)
  line L1 (138, 4) -> (154.5981, 4)
  line L2 (154.5981, 4) -> (161.5263, 0)
  line L3 (161.5263, 0) -> (165, 0)
  line L4 (165, 0) -> (165, 1.5)
  line L5 (165, 1.5) -> (161.9282, 1.5)
  line L6 (161.9282, 1.5) -> (155, 5.5)
  line L7 (155, 5.5) -> (138, 5.5)
  line L8 (138, 5.5) -> (138, 4)
  constraints: 18 end point
revolve "Revolution31" add sketch "Sketch_31" angle 90 about axis through (186, 4, -124) along (0, -1, 0)
sketch "Sketch_32" plane through (186, 0, 0) normal (1, 0, 0) x (0, 0, -1)
  line L0 (-33, 5.5) -> (-33, 4)
  line L1 (-74, 0) -> (-70.5263, 0)
  line L2 (-70.5263, 0) -> (-63.5981, 4)
  line L3 (-63.5981, 4) -> (-47, 4)
  line L4 (-47, 4) -> (-47, 5.5)
  line L5 (-47, 5.5) -> (-64, 5.5)
  line L6 (-64, 5.5) -> (-70.9282, 1.5)
  line L7 (-70.9282, 1.5) -> (-74, 1.5)
  line L8 (-74, 1.5) -> (-74, 0)
  constraints: 18 end point
revolve "Revolution32" add sketch "Sketch_32" angle 90 about axis through (186, 5.5, 33) along (0, 1, 0)
sketch "Sketch_33" plane through (-186, 0, 0) normal (1, 0, 0) x (0, 0, -1)
  line L0 (124, 4) -> (124, 5.5)
  line L1 (138, 4) -> (154.5981, 4)
  line L2 (154.5981, 4) -> (161.5263, 0)
  line L3 (161.5263, 0) -> (165, 0)
  line L4 (165, 0) -> (165, 1.5)
  line L5 (165, 1.5) -> (161.9282, 1.5)
  line L6 (161.9282, 1.5) -> (155, 5.5)
  line L7 (155, 5.5) -> (138, 5.5)
  line L8 (138, 5.5) -> (138, 4)
  constraints: 18 end point
revolve "Revolution33" add sketch "Sketch_33" angle 90 about axis through (-186, 4, -124) along (0, 1, 0)
sketch "Sketch_34" plane through (-186, 0, 0) normal (1, 0, 0) x (0, 0, -1)
  line L0 (-33, 5.5) -> (-33, 4)
  line L1 (-74, 0) -> (-70.5263, 0)
  line L2 (-70.5263, 0) -> (-63.5981, 4)
  line L3 (-63.5981, 4) -> (-47, 4)
  line L4 (-47, 4) -> (-47, 5.5)
  line L5 (-47, 5.5) -> (-64, 5.5)
  line L6 (-64, 5.5) -> (-70.9282, 1.5)
  line L7 (-70.9282, 1.5) -> (-74, 1.5)
  line L8 (-74, 1.5) -> (-74, 0)
  constraints: 18 end point
revolve "Revolution34" add sketch "Sketch_34" angle 90 about axis through (-186, 5.5, 33) along (0, -1, 0)
sketch "Sketch_35" plane through (0, 0, -45.5) normal (0, 0, 1) x (1, 0, 0)
  line L0 (200, 4) -> (216.5981, 4)
  line L1 (216.5981, 4) -> (223.5263, 0)
  line L2 (223.5263, 0) -> (225, 0)
  line L3 (225, 0) -> (225, 1.5)
  line L4 (225, 1.5) -> (223.9282, 1.5)
  line L5 (223.9282, 1.5) -> (217, 5.5)
  line L6 (217, 5.5) -> (200, 5.5)
  line L7 (200, 5.5) -> (200, 4)
  constraints: 16 end point
extrude "Extrusion28" add sketch "Sketch_35" along normal mid plane 157
sketch "Sketch_36" plane through (0, 0, -45.5) normal (0, 0, 1) x (1, 0, 0)
  line L0 (-225, 0) -> (-223.5263, 0)
  line L1 (-223.5263, 0) -> (-216.5981, 4)
  line L2 (-216.5981, 4) -> (-200, 4)
  line L3 (-200, 4) -> (-200, 5.5)
  line L4 (-200, 5.5) -> (-217, 5.5)
  line L5 (-217, 5.5) -> (-223.9282, 1.5)
  line L6 (-223.9282, 1.5) -> (-225, 1.5)
  line L7 (-225, 1.5) -> (-225, 0)
  constraints: 16 end point
extrude "Extrusion29" add sketch "Sketch_36" along normal mid plane 157
sketch "Sketch_37" plane through (0, 5.5, 0) normal (0, 1, 0) x (1, 0, 0)
  arc A0 (-215, -34) -> (-187, -62) centre (-187, -34) ccw
  line L0 (-187, -62) -> (187, -62)
  arc A1 (187, -62) -> (215, -34) centre (187, -34) ccw
  line L1 (215, -34) -> (215, 125)
  arc A2 (215, 125) -> (187, 153) centre (187, 125) ccw
  line L2 (187, 153) -> (-187, 153)
  arc A3 (-187, 153) -> (-215, 125) centre (-187, 125) ccw
  line L3 (-215, 125) -> (-215, -34)
  constraints: 8 end point, 8 point on circle, 4 centre point
extrude "Extrusion30" cut sketch "Sketch_37" against normal blind 1.5
sketch "Sketch_94" plane through (0, 5.5, 0) normal (0, 1, 0) x (1, 0, 0)
  arc A0 (-215, -34) -> (-187, -62) centre (-187, -34) ccw
  line L0 (-187, -62) -> (187, -62)
  arc A1 (187, -62) -> (215, -34) centre (187, -34) ccw
  line L1 (215, -34) -> (215, 125)
  arc A2 (215, 125) -> (187, 153) centre (187, 125) ccw
  line L2 (187, 153) -> (-187, 153)
  arc A3 (-187, 153) -> (-215, 125) centre (-187, 125) ccw
  line L3 (-215, 125) -> (-215, -34)
  circle A4 centre (210, 8.75) radius 2.2
  circle A5 centre (210, 82.25) radius 2.2
  circle A6 centre (168.5, -57) radius 2.2
  circle A7 centre (168.5, 148) radius 2.2
  circle A8 centre (56, -57) radius 2.2
  circle A9 centre (56, 148) radius 2.2
  circle A10 centre (-56, -57) radius 2.2
  circle A11 centre (-56, 148) radius 2.2
  circle A12 centre (-168.5, -57) radius 2.2
  circle A13 centre (-168.5, 148) radius 2.2
  arc A14 (-200, -39) -> (-192, -47) centre (-192, -39) ccw
  line L4 (-192, -47) -> (192, -47)
  arc A15 (192, -47) -> (200, -39) centre (192, -39) ccw
  line L5 (200, -39) -> (200, 130)
  arc A16 (200, 130) -> (192, 138) centre (192, 130) ccw
  line L6 (192, 138) -> (-192, 138)
  arc A17 (-192, 138) -> (-200, 130) centre (-192, 130) ccw
  line L7 (-200, 130) -> (-200, -39)
  circle A18 centre (-210, 8.75) radius 2.2
  circle A19 centre (-210, 82.25) radius 2.2
  constraints: 20 centre point, 16 end point, 16 point on circle
extrude "Extrusion31" add sketch "Sketch_94" against normal blind 1.5
sketch "Sketch_83" plane through (0, 0, 82.5) normal (0, 0, 1) x (1, 0, 0)
  line L0 (298.5, 17.5) -> (278.1, 17.5)
  line L1 (278.1, 17.5) -> (278.1, 20.733)
  line L2 (278.1, 20.733) -> (278.867, 21.5)
  line L3 (278.867, 21.5) -> (293.1, 21.5)
  line L4 (293.1, 21.5) -> (293.1, 23.25)
  line L5 (293.1, 23.25) -> (294, 23.25)
  line L6 (294, 23.25) -> (294, 24.5)
  line L7 (294, 24.5) -> (296.5, 24.5)
  line L8 (296.5, 24.5) -> (297.7, 22.5)
  line L9 (297.7, 22.5) -> (298.5, 22.5)
  line L10 (298.5, 22.5) -> (298.5, 17.5)
  line L11 (298.5, 17.5) -> (278.1, 17.5)
  constraints: 24 end point